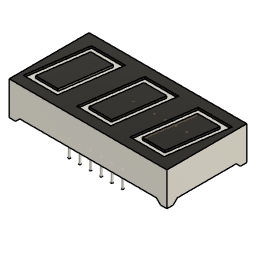
FJ5361BH (Autodesk Fusion 360 design; units mm, degrees)
Autodesk Fusion 360 part; units mm, degrees
sketch "Sketch1" plane through (0, 0, 0) normal (0, 0, 1) x (1, 0, 0)
  line L0 (18.75, -9.5) -> (-18.75, -9.5)
  line L1 (-18.75, -9.5) -> (-18.75, 9.5)
  line L2 (-18.75, 9.5) -> (18.75, 9.5)
  line L3 (18.75, 9.5) -> (18.75, -9.5)
  line L4 (18.75, -9.5) -> (-18.75, 9.5) construction
  line L5 (-18.75, -9.5) -> (18.75, 9.5) construction
  line L6 (0, 9.5) -> (0, -9.5) construction
  line L7 (12.7, 9.5) -> (12.7, -9.5) construction
  line L8 (-12.7, 9.5) -> (-12.7, -9.5) construction
  line L9 (-5.1, -7.1) -> (3, -7.1)
  line L10 (-3.1043, 7.1) -> (4.9957, 7.1)
  line L11 (-5.1, -7.1) -> (-3.1043, 7.1)
  line L12 (3, -7.1) -> (4.9957, 7.1)
  line L13 (-1.9308, 5.75) -> (3.4427, 5.75)
  line L14 (1.8265, -5.75) -> (3.4427, 5.75)
  line L15 (-3.547, -5.75) -> (1.8265, -5.75)
  line L16 (-3.547, -5.75) -> (-1.9308, 5.75)
  line L17 (-17.8, -7.1) -> (-15.8043, 7.1)
  line L18 (-16.247, -5.75) -> (-14.6308, 5.75)
  line L19 (-17.8, -7.1) -> (-9.7, -7.1)
  line L20 (-16.247, -5.75) -> (-10.8735, -5.75)
  line L21 (-10.8735, -5.75) -> (-9.2573, 5.75)
  line L22 (-9.7, -7.1) -> (-7.7043, 7.1)
  line L23 (-14.6308, 5.75) -> (-9.2573, 5.75)
  line L24 (-15.8043, 7.1) -> (-7.7043, 7.1)
  line L25 (7.6, -7.1) -> (9.5957, 7.1)
  line L26 (9.153, -5.75) -> (10.7692, 5.75)
  line L27 (7.6, -7.1) -> (15.7, -7.1)
  line L28 (9.153, -5.75) -> (14.5265, -5.75)
  line L29 (14.5265, -5.75) -> (16.1427, 5.75)
  line L30 (15.7, -7.1) -> (17.6957, 7.1)
  line L31 (10.7692, 5.75) -> (16.1427, 5.75)
  line L32 (9.5957, 7.1) -> (17.6957, 7.1)
  dimension "d1" = 37.5
  dimension "d2" = 19
  dimension "d3" = 12.7
  dimension "d4" = 12.7
  dimension "d5" = 8.1
  dimension "d6" = 3
  dimension "d7" = 2.4
  dimension "d8" = 8.1
  dimension "d9" = 2.4
  dimension "d10" = 82
  dimension "d11" = -1.35
  dimension "d14" = 12.7
  dimension "d15" = 0
  constraint horizontal L0
  constraint perpendicular L0 L1
  constraint parallel L0 L2
  constraint parallel L1 L3
  constraint coincident L4 origin
  constraint coincident L5 origin
  constraint midpoint L2 L6.start
  constraint midpoint L0 L6.end
  constraint coincident L2 L7.start
  constraint coincident L0 L7.end
  constraint perpendicular L0 L7
  constraint coincident L2 L8.start
  constraint coincident L0 L8.end
  constraint perpendicular L0 L8
  constraint perpendicular L6 L9
  constraint perpendicular L6 L10
  measures "d1" distance of L1.end L2.end
  measures "d2" distance of L0.end L1.end
  measures "d3" distance of L6 L8
  measures "d4" distance of L6 L7
  measures "d5" distance of L9.start L9.end
  measures "d6" distance of L6 L9.end
  measures "d7" distance of L0 L9
  measures "d8" distance of L10.start L10.end
  measures "d9" distance of L2 L10
  measures "d10" angle of L9 L11
extrude "Extrude1" add sketch "Sketch1" against normal blind 8 contours L0 L1 L2 L3 | L9 L10 L11 L12 | L13 L14 L15 L16 | L17 L19 L22 L24 | L18 L20 L21 L23 | L25 L27 L30 L32 | L26 L28 L29 L31
extrude "Extrude2" cut sketch "Sketch1" against normal blind 0.5 contours L9 L10 L11 L12 | L17 L19 L22 L24 | L25 L27 L30 L32
sketch "Sketch2" plane through (0, -9.5, 0) normal (0, -1, 0) x (1, 0, 0)
  line L0 (18.75, 0) -> (-18.75, 0)
  line L1 (-18.75, 0) -> (-18.75, -8)
  line L2 (-18.75, -8) -> (18.75, -8)
  line L3 (18.75, -8) -> (18.75, 0)
  line L4 (-17.25, -8) -> (-16.25, -7)
  line L5 (-16.25, -7) -> (16.25, -7)
  line L6 (16.25, -7) -> (17.25, -8)
  dimension "d20" = 1
  dimension "d21" = 1.5
  dimension "d22" = 1.5
  dimension "d23" = 45
  constraint coincident L2 L4.start
  constraint parallel L2 L5
  constraint coincident L2 L6.end
  constraint perpendicular L4 L6
  measures "d20" distance of L2 L5
  measures "d21" distance of L1.end L4.start
  measures "d22" distance of L2.end L6.end
  measures "d23" angle of L2 L6
extrude "Extrude3" cut sketch "Sketch2" against normal up to surface (19 mm away) contours L2 L4 L5 L6
sketch "Sketch3" plane through (-18.75, 0, 0) normal (-1, 0, 0) x (0, -1, 0)
  line L0 (9.5, 0) -> (-9.5, 0)
  line L1 (-9.5, 0) -> (-9.5, -8)
  line L2 (-9.5, -8) -> (9.5, -8)
  line L3 (9.5, -8) -> (9.5, 0)
  line L4 (-8, -8) -> (-7, -7)
  line L5 (-7, -7) -> (7, -7)
  line L6 (7, -7) -> (8, -8)
  dimension "d26" = 45
  dimension "d27" = 1
  dimension "d28" = 1.5
  dimension "d29" = 1.5
  constraint coincident L2 L4.start
  constraint parallel L2 L5
  constraint coincident L2 L6.end
  constraint perpendicular L4 L6
  measures "d26" angle of L2 L6
  measures "d27" distance of L2 L5
  measures "d28" distance of L2.end L6.end
  measures "d29" distance of L1.end L4.start
extrude "Extrude4" cut sketch "Sketch3" against normal up to surface (37.5 mm away) contours L2 L4 L5 L6
sketch "Sketch4" plane through (0, 0, -7) normal (0, 0, -1) x (1, 0, 0)
  line L0 (16.25, 7) -> (16.25, 9.5)
  line L1 (16.25, 9.5) -> (-16.25, 9.5)
  line L2 (-16.25, 9.5) -> (-16.25, 7)
  line L3 (-16.25, 7) -> (-18.75, 7)
  line L4 (-18.75, 7) -> (-18.75, -7)
  line L5 (-18.75, -7) -> (-16.25, -7)
  line L6 (-16.25, -7) -> (-16.25, -9.5)
  line L7 (-16.25, -9.5) -> (16.25, -9.5)
  line L8 (16.25, -9.5) -> (16.25, -7)
  line L9 (16.25, -7) -> (18.75, -7)
  line L10 (18.75, -7) -> (18.75, 7)
  line L11 (18.75, 7) -> (16.25, 7)
  circle A0 centre (-6.35, 7.62) radius 0.255
  circle A1 centre (-3.81, 7.62) radius 0.255
  circle A2 centre (-1.27, 7.62) radius 0.255
  circle A3 centre (1.27, 7.62) radius 0.255
  circle A4 centre (3.81, 7.62) radius 0.255
  circle A5 centre (6.35, 7.62) radius 0.255
  circle A6 centre (-6.35, -7.62) radius 0.255
  circle A7 centre (-3.81, -7.62) radius 0.255
  circle A8 centre (-1.27, -7.62) radius 0.255
  circle A9 centre (1.27, -7.62) radius 0.255
  circle A10 centre (3.81, -7.62) radius 0.255
  circle A11 centre (6.35, -7.62) radius 0.255
  dimension "d32" = 0.51
  dimension "d33" = 6.35
  dimension "d34" = 7.62
  dimension "d37" = 12.7
  dimension "d38" = -15.24
  measures "d32" diameter of A0
  measures "d33" horizontal distance of origin A0.centre
  measures "d34" vertical distance of origin A0.centre
extrude "Extrude5" add sketch "Sketch4" along normal blind 4 contours A0 | A1 | A2 | A3 | A4 | A5 | A6 | A7 | A8 | A9 | A10 | A11
equation "d4 = d3"
equation "d7 = ( ( 19 - 14.2 ) / 2 ) * 1 mm"
equation "d8 = d5"
equation "d9 = d7"
equation "d22 = d21"
equation "d34 = ( 15.24 / 2 ) * 1 mm"
